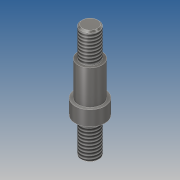
# Autodesk Inventor part: 200-60-DIFFERENTIAL-BAR-02
Saved by Autodesk Inventor 2018.2 (Build 222227000, 227)
## iProperties
Manager: feesmrt
Company: FRANCOR
Part Number: 200-60-DIFFERENTIAL-BAR-02
Material: Edelstahl
Document SubType Name: Modeling
Designer: feesmrt
Density: 8 g/cm^3
Appearance: Halbpoliert
Project: Rescue Robot
Cost Center: -
Engineer: feesmrt
Authority: feesmrt
Description: Differential Stiftverbinder für Kugelgelenk
Stock Number: 200-60-DIFFERENTIAL-BAR-02
Author: feesmrt
Subject: Rescue Robot
Revision Number: 1
Title: Differential Stiftverbinder für Kugelgelenk
Autodesk Inventor part; units mm, degrees
ref_plane "YZ Plane" through (0, 0, 0) normal (1, 0, 0) x (0, 1, 0)
ref_plane "XZ Plane" through (0, 0, 0) normal (0, 1, 0) x (-1, 0, 0)
ref_plane "XY Plane" through (0, 0, 0) normal (0, 0, 1) x (1, 0, 0)
sketch "Skizze1" plane through (0, 0, 0) normal (0, 1, 0) x (-1, 0, 0)
  line L0 (0, -7.7) -> (0, 46.2) projected
  line L1 (-6, 0) -> (1, 0) construction
  line L2 (0, 0) -> (-3, 0)
  line L3 (-3, 0) -> (-3, 12)
  line L4 (-3, 12) -> (-5, 12)
  line L5 (-4, 28.5) -> (-3, 28.5)
  line L6 (-3, 28.5) -> (-3, 38.5)
  line L7 (-3, 38.5) -> (0, 38.5)
  line L8 (0, 38.5) -> (0, 0)
  line L9 (0, 0) -> (0, 38.5)
  line L10 (-5, 12) -> (-5, 17)
  line L11 (-5, 17) -> (-4, 17)
  line L12 (-4, 17) -> (-4, 28.5)
  dimension "d0" = 6
  dimension "d2" = 6
  dimension "d3" = 12
  dimension "d7" = 10
  dimension "d8" = 5
  dimension "d9" = 8
  dimension "d10" = 11.5
  dimension "d12" = 38.5
  constraints: 22 end point, 5 perpendicular, 2 vertical, 1 collinear
  measures "d0" diameter of L3 L0
  measures "d2" diameter of L6 L0
  measures "d3" distance between parallel lines of L1 L4
  measures "d7" diameter of L10 L0
  measures "d8" distance between parallel lines of L11 L4
  measures "d9" diameter of L12 L0
  measures "d10" distance of L11.end L5.start
  measures "d12" distance between parallel lines of L2 L7
revolve "Grundkörper" add sketch "Skizze1" angle 360 about axis through (0, 0, 0) along (0, 0, 1)
thread "M6-1" size "M6x1" class "6g" standard "ANSI Metric M Profile" full length
thread "M6-2" size "M6x1" class "6g" standard "ANSI Metric M Profile" full length
chamfer "Fase_Allgemein" distance 0.5 angle 45 2 edges at (-3, 0, 38.5) (-3, 0, 0)
